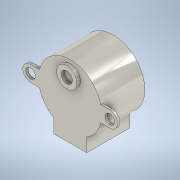
# Autodesk Inventor part: Подставки шаговику
Saved by Autodesk Inventor 2022 (Build 260153000, 153)
## iProperties
Created: 2022-06-07
Part Number: Подставки шаговику
Material: Типовые
Document SubType Name: Modeling
Designer: Admin
Density: 1 g/cm^3
Appearance: По умолчанию
Author: Admin
Autodesk Inventor part; units mm, degrees
ref_plane "YZ Plane" through (0, 0, 0) normal (1, 0, 0) x (0, 1, 0)
ref_plane "XZ Plane" through (0, 0, 0) normal (0, 1, 0) x (-1, 0, 0)
ref_plane "XY Plane" through (0, 0, 0) normal (0, 0, 1) x (1, 0, 0)
sketch "Эскиз1" plane through (0, 0, 0) normal (0, 0, 1) x (1, 0, 0)
  line L0 (13.5554, 3.5) -> (17.5, 3.5)
  line L1 (17.5, -3.5) -> (13.5554, -3.5)
  line L2 (-13.5554, 3.5) -> (-17.5, 3.5)
  line L3 (-17.5, -3.5) -> (-13.5554, -3.5)
  circle A0 centre (-17.5, 0) radius 2.1
  circle A1 centre (17.5, 0) radius 2.1
  arc A2 (17.5, -3.5) -> (17.5, 3.5) centre (17.5, 0) ccw
  arc A3 (-17.5, 3.5) -> (-17.5, -3.5) centre (-17.5, 0) ccw
  circle A4 centre (0, 0) radius 14
  line L4 (-7.3, -11.9461) -> (7.3, -11.9461)
  line L5 (7.3, -11.9461) -> (7.3, -18)
  line L6 (7.3, -18) -> (-7.3, -18)
  line L7 (-7.3, -18) -> (-7.3, -11.9461)
  circle A5 centre (0, 8) radius 4.5
  circle A6 centre (0, 8) radius 2.5
  line L8 (-2, 9.5) -> (2, 9.5)
  line L9 (2, 6.5) -> (-2, 6.5)
  point P0 (0, -11.9461)
  dimension "d8" = 7
  dimension "d9" = 4.2
  dimension "d10" = 7
  dimension "d11" = 7
  dimension "d12" = 7
  dimension "d13" = 35
  dimension "d14" = 28
  dimension "d15" = 14.6
  dimension "d17" = 18
  dimension "d18" = 8
  dimension "d19" = 9
  dimension "d20" = 5
  dimension "d21" = 3
  constraints: 20 end point, 12 point on circle, 7 centre point, 5 parallel, 4 horizontal, 3 coincident, 3 tangent, 2 concentric, 2 equal length, 2 point on line, 2 vertical alignment, 1 equal radius, 1 midpoint, 1 perpendicular
  measures "d8" distance of L0.end L1.start
  measures "d9" diameter of A0
  measures "d10" distance between parallel lines of L3 L2
  measures "d11" distance of L3.end L2.start
  measures "d12" distance of L1.end L0.start
  measures "d13" distance of A0.centre A1.centre
  measures "d14" diameter of A4
  measures "d15" distance of L5.end L6.end
  measures "d17" distance from line of point (0, 0) L6
  measures "d18" distance of A6.centre point (0, 0)
  measures "d19" diameter of A5
  measures "d20" diameter of A6
  measures "d21" distance between parallel lines of L8 L9
extrude "Выдавливание1" add sketch "Эскиз1" against normal blind 19 contours A4 L4 | L5 L6 L7 A4 | A4 L4 | A5 | A6 L9 L8 | L8 A6 | A6 L9
extrude "Выдавливание2" add sketch "Эскиз1" along normal blind 1.5 contours A5 | A6 L9 L8 | L8 A6 | A6 L9
extrude "Выдавливание3" add sketch "Эскиз1" against normal blind 1 contours L0 A2 L1 A4 | A4 L3 A3 L2
sketch "Эскиз3" plane through (0, 0, 0) normal (0, 0, 1) x (1, 0, 0)
  circle A0 centre (0, 8) radius 2.5
  arc A1 (2, 6.5) -> (2, 9.5) centre (0, 8) ccw projected
  point P0 (0, 0)
  constraints: 2 concentric, 1 centre point
extrude "Выдавливание5" cut sketch "Эскиз1" along normal blind 10 contours A6 L9 L8 | L8 A6 | A6 L9
